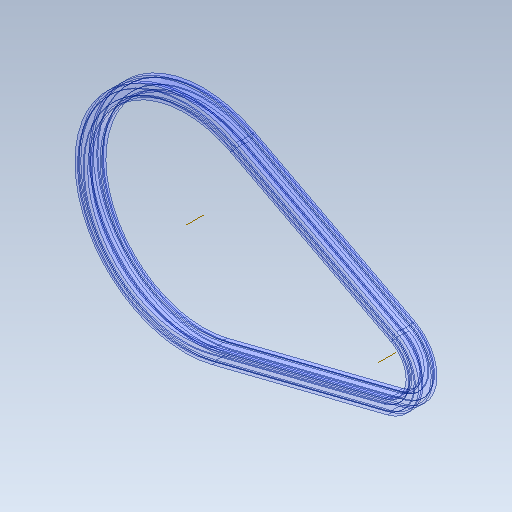
# Autodesk Inventor part: Cadena de rodillos
Saved by Autodesk Inventor 2020 (Build 240168000, 168)
## iProperties
Created: 2021-01-16
Part Number: Cadena de rodillos
Material: Generic
Document SubType Name: Modeling
Designer: pc-home
Density: 1 g/cm^3
Appearance: Clear - Blue
CustomPartVersion: 1
Author: pc-home
Autodesk Inventor part; units mm, degrees
ref_plane "Plano de trabajo2" through (0, 0, 0) normal (-1, 0, 0) x (0, 0, 1)
ref_plane "Plano de trabajo3" through (-505.7662, 59.9289, 0) normal (0.986769, 0.1621325, 0) x (0, 0, 1)
sketch "Trayectoria" plane through (0, 0, 0) normal (0, 0, 1) x (1, 0, 0)
  arc A0 (22.346, -88.8588) -> (42.4936, 81.1758) centre (0, 0) ccw
  arc A1 (-379.1125, 301.8764) -> (-439.1632, -204.9179) centre (-505.7662, 59.9289) ccw
  line L0 (-379.1125, 301.8764) -> (42.4936, 81.1758)
  line L1 (22.346, -88.8588) -> (-439.1632, -204.9179)
  dimension "d31" = 33.4
  constraints: 4 end point, 4 point on circle, 2 centre point
ref_plane "Plano de sección" through (42.4936, 81.1758, 0) normal (-0.8859531, 0.4637749, 0) x (0, 0, 1)
sketch "Boceto de sección" plane through (42.4936, 81.1758, 0) normal (-0.8859531, 0.4637749, 0) x (0, 0, 1)
  line L0 (-26.7, -7.315) -> (26.7, -7.315)
  line L1 (26.7, -7.315) -> (26.7, 7.315)
  line L2 (26.7, 7.315) -> (-26.7, 7.315)
  line L3 (-26.7, 7.315) -> (-26.7, -7.315)
  line L4 (-12.7, -12.7) -> (12.7, -12.7)
  line L5 (12.7, -12.7) -> (12.7, 12.7)
  line L6 (12.7, 12.7) -> (-12.7, 12.7)
  line L7 (-12.7, 12.7) -> (-12.7, -12.7)
  line L8 (-12.7, 0) -> (12.7, 0) construction
  line L9 (-23.9, -16.7) -> (-12.7, -16.7)
  line L10 (-12.7, -16.7) -> (-12.7, 16.7)
  line L11 (-12.7, 16.7) -> (-23.9, 16.7)
  line L12 (-23.9, 16.7) -> (-23.9, -16.7)
  line L13 (12.7, -16.7) -> (23.9, -16.7)
  line L14 (23.9, -16.7) -> (23.9, 16.7)
  line L15 (23.9, 16.7) -> (12.7, 16.7)
  line L16 (12.7, 16.7) -> (12.7, -16.7)
  line L17 (-26.7, 0) -> (26.7, 0) construction
  point P0 (0, 0)
  point P1 (0, 0)
  dimension "d21" = 14.63
  dimension "d22" = 25.4
  dimension "d23" = 25.4
  dimension "d24" = 11.2
  dimension "d31" = 33.4
  dimension "d32" = 53.4
  constraints: 36 end point, 8 midpoint, 8 parallel, 4 horizontal, 4 perpendicular, 3 collinear, 1 coincident, 1 other
  measures "d21" distance between parallel lines of L2 L0
  measures "d22" distance between parallel lines of L6 L4
  measures "d23" distance between parallel lines of L5 L7
  measures "d24" distance between parallel lines of L12 L10
  measures "d31" distance between parallel lines of L11 L9
  measures "d32" distance between parallel lines of L1 L3
sweep "Sólido" add profiles "Boceto de sección" path "Trayectoria"
pattern_of_one "Strand Pattern"
equation "\"d21\" = da_d2"
equation "\"d22\" = da_d1"
equation "\"d23\" = da_b1"
equation "\"d24\" = da_t1 + da_t2"
equation "\"d30\" = da_pt"
equation "\"da_p\" = 38.1"
equation "\"da_b1\" = 25.4"
equation "\"da_h2\" = 33.4"
equation "\"da_h3\" = 33.4"
equation "\"da_d1\" = 25.4"
equation "\"da_d2\" = 14.63"
equation "\"da_pt\" = 48.36"
equation "\"da_b\" = 53.4"
equation "\"da_t1\" = 6"
equation "\"da_t2\" = 5.2"
body "Solid1"
